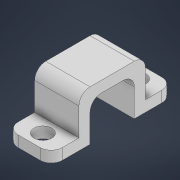
# Autodesk Inventor part: Kabelhalterung
Saved by Autodesk Inventor 2021 (Build 250183000, 183)
## iProperties
Created: 2021-02-05
Part Number: Kabelhalterung
Material: Generisch
Document SubType Name: Modeling
Designer: laure
Density: 1 g/cm^3
Appearance: Vorgabe
Author: laure
Autodesk Inventor part; units mm, degrees
ref_plane "YZ Plane" through (0, 0, 0) normal (1, 0, 0) x (0, 1, 0)
ref_plane "XZ Plane" through (0, 0, 0) normal (0, 1, 0) x (-1, 0, 0)
ref_plane "XY Plane" through (0, 0, 0) normal (0, 0, 1) x (1, 0, 0)
sketch "Skizze1" plane through (0, 0, 0) normal (0, 1, 0) x (-1, 0, 0)
  line L0 (4, -6) -> (-4, -6)
  line L1 (-4, -6) -> (-4, 6)
  line L2 (-4, 6) -> (4, 6)
  line L3 (4, 6) -> (4, -6)
  line L4 (0, -8.4) -> (0, 8.4) projected
  line L5 (-5.6, 0) -> (5.6, 0) projected
  point P0 (0, 0)
  dimension "d0" = 8
  dimension "d1" = 12
  constraints: 8 end point, 2 parallel, 1 horizontal, 1 perpendicular, 2 other
  measures "d0" distance of L1.end L2.end
  measures "d1" distance of L0.end L1.end
extrude "Extrusion1" add sketch "Skizze1" along normal mid plane 2
sketch "Skizze2" plane through (0, -1, 0) normal (0, -1, 0) x (1, 0, 0)
  line L0 (-4, -6) -> (-4, 6) projected
  line L1 (4, 6) -> (4, -6) projected
  line L2 (-4, -6) -> (4, -6)
  line L3 (4, -6) -> (4, -4)
  line L4 (4, -4) -> (-4, -4)
  line L5 (-4, -4) -> (-4, -6)
  line L6 (-4, 6) -> (4, 6)
  line L7 (4, 6) -> (4, 4)
  line L8 (4, 4) -> (-4, 4)
  line L9 (-4, 4) -> (-4, 6)
  point P0 (0, 0)
  dimension "d4" = 2
  dimension "d5" = 2
  constraints: 16 end point, 4 parallel, 2 horizontal, 2 perpendicular, 2 point on line
  measures "d4" distance of L3.end L2.end
  measures "d5" distance of L6.end L7.end
extrude "Extrusion2" add sketch "Skizze2" along normal blind 7 contours L0 L4 L1 L2 | L0 L6 L1 L8
sketch "Skizze3" plane through (4, 1, 6) normal (1, 0, 0) x (0, 0, -1)
  line L0 (2, -9) -> (0, -9) projected
  line L1 (0, -9) -> (-5, -9)
  line L2 (-5, -9) -> (-5, -7)
  line L3 (-5, -7) -> (0, -7)
  line L4 (0, -7) -> (0, -9)
  line L5 (12, -9) -> (10, -9) projected
  line L6 (12, -9) -> (17, -9)
  line L7 (17, -9) -> (17, -7)
  line L8 (17, -7) -> (12, -7)
  line L9 (12, -7) -> (12, -9)
  point P0 (6, -1)
  dimension "d8" = 5
  dimension "d9" = 2
  dimension "d10" = 5
  dimension "d11" = 2
  constraints: 16 end point, 4 parallel, 2 horizontal, 2 perpendicular
  measures "d8" distance of L2.end L3.end
  measures "d9" distance of L1.end L2.end
  measures "d10" distance of L8.end L7.end
  measures "d11" distance of L7.end L6.end
extrude "Extrusion3" add sketch "Skizze3" against normal blind 8
sketch "Skizze4" plane through (4, -6, 11) normal (0, 1, 0) x (1, 0, 0)
  circle A0 centre (-4, 2.5) radius 1.6
  line L0 (0, 5) -> (0, 0) projected
  line L1 (0, 0) -> (-8, 0) projected
  circle A1 centre (-4, 19.5) radius 1.6
  line L2 (0, 22) -> (0, 17) projected
  line L3 (0, 22) -> (-8, 22) projected
  point P0 (-4, 11)
  dimension "d14" = 3.2
  dimension "d15" = 4
  dimension "d16" = 2.5
  dimension "d17" = 3.2
  dimension "d18" = 4
  dimension "d19" = 2.5
  constraints: 2 centre point
  measures "d14" diameter of A0
  measures "d15" distance from line of L0 A0.centre
  measures "d16" distance from line of L1 A0.centre
  measures "d17" diameter of A1
  measures "d18" distance from line of L2 A1.centre
  measures "d19" distance from line of L3 A1.centre
extrude "Extrusion4" cut sketch "Skizze4" against normal up to surface (2 mm away)
fillet "Rundung1" radius 2 8 edges at (0, 1, 6) (0, 1, -6) (0, -1, 4) (0, -1, -4) (-4, -7, 11) (4, -7, 11) (4, -7, -11) (-4, -7, -11)
